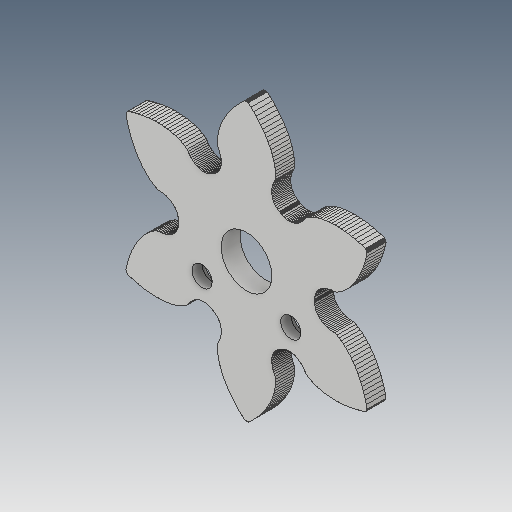
# Autodesk Inventor part: m5-6(dis0.4)
Saved by Autodesk Inventor 2019.4 (Build 234330000, 330)
## iProperties
Created: 2019-06-11
Part Number: m5-6(dis0.4)
Material: Generic
Document SubType Name: Modeling
Designer: AzLIer
Density: 1 g/cm^3
Appearance: Default
Mass: 2.28533 g
Surface Area: 21.9725 cm^2
Volume: 2.28533 cm^3
Autodesk Inventor part; units mm, degrees
ref_plane "YZ Plane" through (0, 0, 0) normal (1, 0, 0) x (0, 1, 0)
ref_plane "XZ Plane" through (0, 0, 0) normal (0, 1, 0) x (-1, 0, 0)
ref_plane "XY Plane" through (0, 0, 0) normal (0, 0, 1) x (1, 0, 0)
sketch "スケッチ1" plane through (0, 0, 0) normal (0, 0, 1) x (1, 0, 0)
  circle A0 centre (0, 0) radius 15 construction
  line L0 (-18, 0) -> (18, 0) construction
  line L1 (0, -18) -> (0, 18) construction
  line L2 (10.75, 0) -> (10.7499, 0.0461)
  line L3 (10.7499, 0.0461) -> (10.7496, 0.0922)
  line L4 (10.7496, 0.0922) -> (10.7491, 0.1384)
  line L5 (10.7491, 0.1384) -> (10.7484, 0.1845)
  line L6 (10.7484, 0.1845) -> (10.7475, 0.2306)
  line L7 (10.7475, 0.2306) -> (10.7652, 0.5329)
  line L8 (10.7652, 0.5329) -> (10.8097, 0.7549)
  line L9 (10.8097, 0.7549) -> (10.869, 0.9963)
  line L10 (10.869, 0.9963) -> (10.9454, 1.1976)
  line L11 (10.9454, 1.1976) -> (11.037, 1.3769)
  line L12 (11.037, 1.3769) -> (11.1429, 1.5397)
  line L13 (11.1429, 1.5397) -> (11.2607, 1.6996)
  line L14 (11.2607, 1.6996) -> (11.39, 1.856)
  line L15 (11.39, 1.856) -> (11.5328, 1.9955)
  line L16 (11.5328, 1.9955) -> (11.6888, 2.1189)
  line L17 (11.6888, 2.1189) -> (11.8558, 2.239)
  line L18 (11.8558, 2.239) -> (12.034, 2.3529)
  line L19 (12.034, 2.3529) -> (12.2259, 2.4472)
  line L20 (12.2259, 2.4472) -> (12.4297, 2.5309)
  line L21 (12.4297, 2.5309) -> (12.6434, 2.613)
  line L22 (12.6434, 2.613) -> (12.8716, 2.6699)
  line L23 (12.8716, 2.6699) -> (13.1096, 2.7237)
  line L24 (13.1096, 2.7237) -> (13.3595, 2.7636)
  line L25 (13.3595, 2.7636) -> (13.6235, 2.7775)
  line L26 (13.6235, 2.7775) -> (13.8941, 2.7998)
  line L27 (13.8941, 2.7998) -> (14.254, 2.9465)
  line L28 (14.254, 2.9465) -> (14.6036, 3.1397)
  line L29 (14.6036, 3.1397) -> (14.9447, 3.367)
  line L30 (14.9447, 3.367) -> (15.2773, 3.6237)
  line L31 (15.2773, 3.6237) -> (15.6013, 3.9073)
  line L32 (15.6013, 3.9073) -> (15.9161, 4.216)
  line L33 (15.9161, 4.216) -> (16.2214, 4.5483)
  line L34 (16.2214, 4.5483) -> (16.5165, 4.9034)
  line L35 (16.5165, 4.9034) -> (16.8007, 5.2802)
  line L36 (16.8007, 5.2802) -> (17.0734, 5.678)
  line L37 (17.0734, 5.678) -> (17.334, 6.0961)
  line L38 (17.334, 6.0961) -> (17.5819, 6.5338)
  line L39 (17.5819, 6.5338) -> (17.8162, 6.9906)
  line L40 (17.8162, 6.9906) -> (18.0365, 7.4658)
  line L41 (18.0365, 7.4658) -> (18.2419, 7.9587)
  line L42 (18.2419, 7.9587) -> (18.4319, 8.469)
  line L43 (18.4319, 8.469) -> (18.6058, 8.9958)
  line L44 (18.6058, 8.9958) -> (18.7629, 9.5386)
  line L45 (18.7629, 9.5386) -> (18.9026, 10.0969)
  line L46 (18.9026, 10.0969) -> (19.0243, 10.6699)
  line L47 (19.0243, 10.6699) -> (18.9976, 10.7173)
  line L48 (18.9976, 10.7173) -> (18.9709, 10.7646)
  line L49 (18.9709, 10.7646) -> (18.944, 10.8118)
  line L50 (18.944, 10.8118) -> (18.917, 10.859)
  line L51 (18.917, 10.859) -> (18.8899, 10.9061)
  line L52 (10.75, 0) -> (10.7499, -0.0461)
  line L53 (10.7499, -0.0461) -> (10.7496, -0.0922)
  line L54 (10.7496, -0.0922) -> (10.7491, -0.1384)
  line L55 (10.7491, -0.1384) -> (10.7484, -0.1845)
  line L56 (10.7484, -0.1845) -> (10.7475, -0.2306)
  line L57 (10.7475, -0.2306) -> (10.7652, -0.5329)
  line L58 (10.7652, -0.5329) -> (10.8097, -0.7549)
  line L59 (10.8097, -0.7549) -> (10.869, -0.9963)
  line L60 (10.869, -0.9963) -> (10.9454, -1.1976)
  line L61 (10.9454, -1.1976) -> (11.037, -1.3769)
  line L62 (11.037, -1.3769) -> (11.1429, -1.5397)
  line L63 (11.1429, -1.5397) -> (11.2607, -1.6996)
  line L64 (11.2607, -1.6996) -> (11.39, -1.856)
  line L65 (11.39, -1.856) -> (11.5328, -1.9955)
  line L66 (11.5328, -1.9955) -> (11.6888, -2.1189)
  line L67 (11.6888, -2.1189) -> (11.8558, -2.239)
  line L68 (11.8558, -2.239) -> (12.034, -2.3529)
  line L69 (12.034, -2.3529) -> (12.2259, -2.4472)
  line L70 (12.2259, -2.4472) -> (12.4297, -2.5309)
  line L71 (12.4297, -2.5309) -> (12.6434, -2.613)
  line L72 (12.6434, -2.613) -> (12.8716, -2.6699)
  line L73 (12.8716, -2.6699) -> (13.1096, -2.7237)
  line L74 (13.1096, -2.7237) -> (13.3595, -2.7636)
  line L75 (13.3595, -2.7636) -> (13.6235, -2.7775)
  line L76 (13.6235, -2.7775) -> (13.8941, -2.7998)
  line L77 (13.8941, -2.7998) -> (14.254, -2.9465)
  line L78 (14.254, -2.9465) -> (14.6036, -3.1397)
  line L79 (14.6036, -3.1397) -> (14.9447, -3.367)
  line L80 (14.9447, -3.367) -> (15.2773, -3.6237)
  line L81 (15.2773, -3.6237) -> (15.6013, -3.9073)
  line L82 (15.6013, -3.9073) -> (15.9161, -4.216)
  line L83 (15.9161, -4.216) -> (16.2214, -4.5483)
  line L84 (16.2214, -4.5483) -> (16.5165, -4.9034)
  line L85 (16.5165, -4.9034) -> (16.8007, -5.2802)
  line L86 (16.8007, -5.2802) -> (17.0734, -5.678)
  line L87 (17.0734, -5.678) -> (17.334, -6.0961)
  line L88 (17.334, -6.0961) -> (17.5819, -6.5338)
  line L89 (17.5819, -6.5338) -> (17.8162, -6.9906)
  line L90 (17.8162, -6.9906) -> (18.0365, -7.4658)
  line L91 (18.0365, -7.4658) -> (18.2419, -7.9587)
  line L92 (18.2419, -7.9587) -> (18.4319, -8.469)
  line L93 (18.4319, -8.469) -> (18.6058, -8.9958)
  line L94 (18.6058, -8.9958) -> (18.7629, -9.5386)
  line L95 (18.7629, -9.5386) -> (18.9026, -10.0969)
  line L96 (18.9026, -10.0969) -> (19.0243, -10.6699)
  line L97 (19.0243, -10.6699) -> (18.9976, -10.7173)
  line L98 (18.9976, -10.7173) -> (18.9709, -10.7646)
  line L99 (18.9709, -10.7646) -> (18.944, -10.8118)
  line L100 (18.944, -10.8118) -> (18.917, -10.859)
  line L101 (18.917, -10.859) -> (18.8899, -10.9061)
  line L102 (5.335, 9.3327) -> (5.2949, 9.3556)
  line L103 (5.2949, 9.3556) -> (5.2547, 9.3782)
  line L104 (4.238, 10.4198) -> (4.1585, 10.6018)
  line L105 (4.3261, 10.2467) -> (4.238, 10.4198)
  line L106 (4.4355, 10.0778) -> (4.3261, 10.2467)
  line L107 (4.5717, 9.9109) -> (4.4355, 10.0778)
  line L108 (4.751, 9.7389) -> (4.5717, 9.9109)
  line L109 (4.9211, 9.5894) -> (4.751, 9.7389)
  line L110 (5.1741, 9.4229) -> (4.9211, 9.5894)
  line L111 (5.2144, 9.4006) -> (5.1741, 9.4229)
  line L112 (5.2547, 9.3782) -> (5.2144, 9.4006)
  line L113 (4.1585, 10.6018) -> (4.0877, 10.792)
  line L114 (4.0877, 10.792) -> (4.0382, 10.9854)
  line L115 (4.0382, 10.9854) -> (4.0094, 11.1823)
  line L116 (4.0094, 11.1823) -> (3.9889, 11.3869)
  line L117 (3.9889, 11.3869) -> (3.9793, 11.5982)
  line L118 (3.9793, 11.5982) -> (3.9936, 11.8115)
  line L119 (3.9936, 11.8115) -> (4.023, 12.0299)
  line L120 (4.023, 12.0299) -> (4.0588, 12.2559)
  line L121 (4.1236, 12.4821) -> (4.196, 12.7151)
  line L122 (4.196, 12.7151) -> (4.2864, 12.9515)
  line L123 (4.2864, 12.9515) -> (4.4064, 13.187)
  line L124 (4.4064, 13.187) -> (4.5223, 13.4326)
  line L125 (4.5223, 13.4326) -> (4.5752, 13.8176)
  line L126 (4.5752, 13.8176) -> (4.5827, 14.217)
  line L127 (4.0588, 12.2559) -> (4.1236, 12.4821)
  line L128 (4.5827, 14.217) -> (4.5564, 14.626)
  line L129 (4.5564, 14.626) -> (4.5004, 15.0424)
  line L130 (4.5004, 15.0424) -> (4.4168, 15.4648)
  line L131 (4.4168, 15.4648) -> (4.3069, 15.8918)
  line L132 (4.3069, 15.8918) -> (4.1717, 16.3223)
  line L133 (4.1717, 16.3223) -> (4.0118, 16.7553)
  line L134 (4.0118, 16.7553) -> (3.8276, 17.1899)
  line L135 (3.8276, 17.1899) -> (3.6194, 17.625)
  line L136 (3.6194, 17.625) -> (3.3877, 18.0598)
  line L137 (3.3877, 18.0598) -> (3.1325, 18.4933)
  line L138 (3.1325, 18.4933) -> (2.8541, 18.9246)
  line L139 (2.8541, 18.9246) -> (2.5527, 19.3529)
  line L140 (2.5527, 19.3529) -> (2.2285, 19.7773)
  line L141 (2.2285, 19.7773) -> (1.8816, 20.197)
  line L142 (1.8816, 20.197) -> (1.5123, 20.611)
  line L143 (1.5123, 20.611) -> (1.1207, 21.0184)
  line L144 (1.1207, 21.0184) -> (0.7071, 21.4186)
  line L145 (0.2717, 21.8105) -> (0.2174, 21.8111)
  line L146 (0.2174, 21.8111) -> (0.163, 21.8116)
  line L147 (0.163, 21.8116) -> (0.1087, 21.8119)
  line L148 (0.1087, 21.8119) -> (0.0543, 21.8121)
  line L149 (0.0543, 21.8121) -> (0, 21.8122)
  line L150 (0.7071, 21.4186) -> (0.2717, 21.8105)
  line L151 (5.375, 9.3098) -> (5.335, 9.3327)
  line L152 (5.375, 9.3098) -> (5.4149, 9.2866)
  line L153 (5.4149, 9.2866) -> (5.4547, 9.2633)
  line L154 (5.4547, 9.2633) -> (5.4944, 9.2398)
  line L155 (5.4944, 9.2398) -> (5.534, 9.2162)
  line L156 (5.534, 9.2162) -> (5.5735, 9.1923)
  line L157 (5.5735, 9.1923) -> (5.8441, 9.0565)
  line L158 (5.8441, 9.0565) -> (6.0586, 8.984)
  line L159 (6.2973, 8.9146) -> (6.5098, 8.8802)
  line L160 (6.5098, 8.8802) -> (6.7109, 8.8699)
  line L161 (6.7109, 8.8699) -> (6.9048, 8.8802)
  line L162 (6.0586, 8.984) -> (6.2973, 8.9146)
  line L163 (6.9048, 8.8802) -> (7.1022, 8.9022)
  line L164 (7.1022, 8.9022) -> (7.3024, 8.936)
  line L165 (7.3024, 8.936) -> (7.4945, 8.9899)
  line L166 (7.4945, 8.9899) -> (7.6794, 9.0634)
  line L167 (7.6794, 9.0634) -> (7.8669, 9.1479)
  line L168 (7.8669, 9.1479) -> (8.0546, 9.2453)
  line L169 (8.0546, 9.2453) -> (8.2323, 9.3643)
  line L170 (8.2323, 9.3643) -> (8.4067, 9.499)
  line L171 (8.4067, 9.499) -> (8.5846, 9.643)
  line L172 (8.5846, 9.643) -> (8.748, 9.8122)
  line L173 (8.748, 9.8122) -> (8.9136, 9.9914)
  line L174 (8.9136, 9.9914) -> (9.0731, 10.1878)
  line L175 (9.2171, 10.4095) -> (9.3718, 10.6328)
  line L176 (9.3718, 10.6328) -> (9.6788, 10.8711)
  line L177 (9.0731, 10.1878) -> (9.2171, 10.4095)
  line L178 (9.6788, 10.8711) -> (10.0209, 11.0772)
  line L179 (10.0209, 11.0772) -> (10.3882, 11.259)
  line L180 (10.3882, 11.259) -> (10.7769, 11.4187)
  line L181 (10.7769, 11.4187) -> (11.1845, 11.5574)
  line L182 (11.1845, 11.5574) -> (11.6092, 11.6758)
  line L183 (11.6092, 11.6758) -> (12.0497, 11.774)
  line L184 (12.0497, 11.774) -> (12.5047, 11.852)
  line L185 (17.0935, 11.6152) -> (17.6421, 11.4798)
  line L186 (17.6421, 11.4798) -> (18.1955, 11.3217)
  line L187 (18.1955, 11.3217) -> (18.7526, 11.1405)
  line L188 (18.7526, 11.1405) -> (18.7803, 11.0938)
  line L189 (18.7803, 11.0938) -> (18.8079, 11.047)
  line L190 (18.8079, 11.047) -> (18.8353, 11.0001)
  line L191 (18.8353, 11.0001) -> (18.8627, 10.9531)
  line L192 (18.8627, 10.9531) -> (18.8899, 10.9061)
  line L193 (12.9731, 11.9097) -> (13.454, 11.947)
  line L194 (13.454, 11.947) -> (13.9464, 11.9637)
  line L195 (13.9464, 11.9637) -> (14.4494, 11.9594)
  line L196 (14.4494, 11.9594) -> (14.9621, 11.934)
  line L197 (14.9621, 11.934) -> (15.4838, 11.8872)
  line L198 (15.4838, 11.8872) -> (16.0134, 11.8186)
  line L199 (16.0134, 11.8186) -> (16.5503, 11.728)
  line L200 (16.5503, 11.728) -> (17.0935, 11.6152)
  line L201 (12.5047, 11.852) -> (12.9731, 11.9097)
  line L202 (-5.4149, 9.2866) -> (-5.4547, 9.2633)
  line L203 (-5.4547, 9.2633) -> (-5.4944, 9.2398)
  line L204 (-6.9048, 8.8802) -> (-7.1022, 8.9022)
  line L205 (-6.7109, 8.8699) -> (-6.9048, 8.8802)
  line L206 (-6.5098, 8.8802) -> (-6.7109, 8.8699)
  line L207 (-6.2973, 8.9146) -> (-6.5098, 8.8802)
  line L208 (-6.0586, 8.984) -> (-6.2973, 8.9146)
  line L209 (-5.8441, 9.0565) -> (-6.0586, 8.984)
  line L210 (-5.5735, 9.1923) -> (-5.8441, 9.0565)
  line L211 (-5.534, 9.2162) -> (-5.5735, 9.1923)
  line L212 (-5.4944, 9.2398) -> (-5.534, 9.2162)
  line L213 (-7.1022, 8.9022) -> (-7.3024, 8.936)
  line L214 (-7.3024, 8.936) -> (-7.4945, 8.9899)
  line L215 (-7.4945, 8.9899) -> (-7.6794, 9.0634)
  line L216 (-7.6794, 9.0634) -> (-7.8669, 9.1479)
  line L217 (-7.8669, 9.1479) -> (-8.0546, 9.2453)
  line L218 (-8.0546, 9.2453) -> (-8.2323, 9.3643)
  line L219 (-8.2323, 9.3643) -> (-8.4067, 9.499)
  line L220 (-8.4067, 9.499) -> (-8.5846, 9.643)
  line L221 (-8.748, 9.8122) -> (-8.9136, 9.9914)
  line L222 (-8.9136, 9.9914) -> (-9.0731, 10.1878)
  line L223 (-9.0731, 10.1878) -> (-9.2171, 10.4095)
  line L224 (-9.2171, 10.4095) -> (-9.3718, 10.6328)
  line L225 (-9.3718, 10.6328) -> (-9.6788, 10.8711)
  line L226 (-9.6788, 10.8711) -> (-10.0209, 11.0772)
  line L227 (-8.5846, 9.643) -> (-8.748, 9.8122)
  line L228 (-10.0209, 11.0772) -> (-10.3882, 11.259)
  line L229 (-10.3882, 11.259) -> (-10.7769, 11.4187)
  line L230 (-10.7769, 11.4187) -> (-11.1845, 11.5574)
  line L231 (-11.1845, 11.5574) -> (-11.6092, 11.6758)
  line L232 (-11.6092, 11.6758) -> (-12.0497, 11.774)
  line L233 (-12.0497, 11.774) -> (-12.5047, 11.852)
  line L234 (-12.5047, 11.852) -> (-12.9731, 11.9097)
  line L235 (-12.9731, 11.9097) -> (-13.454, 11.947)
  line L236 (-13.454, 11.947) -> (-13.9464, 11.9637)
  line L237 (-13.9464, 11.9637) -> (-14.4494, 11.9594)
  line L238 (-14.4494, 11.9594) -> (-14.9621, 11.934)
  line L239 (-14.9621, 11.934) -> (-15.4838, 11.8872)
  line L240 (-15.4838, 11.8872) -> (-16.0134, 11.8186)
  line L241 (-16.0134, 11.8186) -> (-16.5503, 11.728)
  line L242 (-16.5503, 11.728) -> (-17.0935, 11.6152)
  line L243 (-17.0935, 11.6152) -> (-17.6421, 11.4798)
  line L244 (-17.6421, 11.4798) -> (-18.1955, 11.3217)
  line L245 (-18.7526, 11.1405) -> (-18.7803, 11.0938)
  line L246 (-18.7803, 11.0938) -> (-18.8079, 11.047)
  line L247 (-18.8079, 11.047) -> (-18.8353, 11.0001)
  line L248 (-18.8353, 11.0001) -> (-18.8627, 10.9531)
  line L249 (-18.8627, 10.9531) -> (-18.8899, 10.9061)
  line L250 (-18.1955, 11.3217) -> (-18.7526, 11.1405)
  line L251 (-5.375, 9.3098) -> (-5.4149, 9.2866)
  line L252 (-5.375, 9.3098) -> (-5.335, 9.3327)
  line L253 (-5.335, 9.3327) -> (-5.2949, 9.3556)
  line L254 (-5.2949, 9.3556) -> (-5.2547, 9.3782)
  line L255 (-5.2547, 9.3782) -> (-5.2144, 9.4006)
  line L256 (-5.2144, 9.4006) -> (-5.1741, 9.4229)
  line L257 (-5.1741, 9.4229) -> (-4.9211, 9.5894)
  line L258 (-4.9211, 9.5894) -> (-4.751, 9.7389)
  line L259 (-4.5717, 9.9109) -> (-4.4355, 10.0778)
  line L260 (-4.4355, 10.0778) -> (-4.3261, 10.2467)
  line L261 (-4.3261, 10.2467) -> (-4.238, 10.4198)
  line L262 (-4.751, 9.7389) -> (-4.5717, 9.9109)
  line L263 (-4.238, 10.4198) -> (-4.1585, 10.6018)
  line L264 (-4.1585, 10.6018) -> (-4.0877, 10.792)
  line L265 (-4.0877, 10.792) -> (-4.0382, 10.9854)
  line L266 (-4.0382, 10.9854) -> (-4.0094, 11.1823)
  line L267 (-4.0094, 11.1823) -> (-3.9889, 11.3869)
  line L268 (-3.9889, 11.3869) -> (-3.9793, 11.5982)
  line L269 (-3.9793, 11.5982) -> (-3.9936, 11.8115)
  line L270 (-3.9936, 11.8115) -> (-4.023, 12.0299)
  line L271 (-4.023, 12.0299) -> (-4.0588, 12.2559)
  line L272 (-4.0588, 12.2559) -> (-4.1236, 12.4821)
  line L273 (-4.1236, 12.4821) -> (-4.196, 12.7151)
  line L274 (-4.196, 12.7151) -> (-4.2864, 12.9515)
  line L275 (-4.4064, 13.187) -> (-4.5223, 13.4326)
  line L276 (-4.5223, 13.4326) -> (-4.5752, 13.8176)
  line L277 (-4.2864, 12.9515) -> (-4.4064, 13.187)
  line L278 (-4.5752, 13.8176) -> (-4.5827, 14.217)
  line L279 (-4.5827, 14.217) -> (-4.5564, 14.626)
  line L280 (-4.5564, 14.626) -> (-4.5004, 15.0424)
  line L281 (-4.5004, 15.0424) -> (-4.4168, 15.4648)
  line L282 (-4.4168, 15.4648) -> (-4.3069, 15.8918)
  line L283 (-4.3069, 15.8918) -> (-4.1717, 16.3223)
  line L284 (-4.1717, 16.3223) -> (-4.0118, 16.7553)
  line L285 (-1.5123, 20.611) -> (-1.1207, 21.0184)
  line L286 (-1.1207, 21.0184) -> (-0.7071, 21.4186)
  line L287 (-0.7071, 21.4186) -> (-0.2717, 21.8105)
  line L288 (-0.2717, 21.8105) -> (-0.2174, 21.8111)
  line L289 (-0.2174, 21.8111) -> (-0.163, 21.8116)
  line L290 (-0.163, 21.8116) -> (-0.1087, 21.8119)
  line L291 (-0.1087, 21.8119) -> (-0.0543, 21.8121)
  line L292 (-0.0543, 21.8121) -> (0, 21.8122)
  line L293 (-3.8276, 17.1899) -> (-3.6194, 17.625)
  line L294 (-3.6194, 17.625) -> (-3.3877, 18.0598)
  line L295 (-3.3877, 18.0598) -> (-3.1325, 18.4933)
  line L296 (-3.1325, 18.4933) -> (-2.8541, 18.9246)
  line L297 (-2.8541, 18.9246) -> (-2.5527, 19.3529)
  line L298 (-2.5527, 19.3529) -> (-2.2285, 19.7773)
  line L299 (-2.2285, 19.7773) -> (-1.8816, 20.197)
  line L300 (-1.8816, 20.197) -> (-1.5123, 20.611)
  line L301 (-4.0118, 16.7553) -> (-3.8276, 17.1899)
  line L302 (-10.7499, -0.0461) -> (-10.7496, -0.0922)
  line L303 (-10.7496, -0.0922) -> (-10.7491, -0.1384)
  line L304 (-11.1429, -1.5397) -> (-11.2607, -1.6996)
  line L305 (-11.037, -1.3769) -> (-11.1429, -1.5397)
  line L306 (-10.9454, -1.1976) -> (-11.037, -1.3769)
  line L307 (-10.869, -0.9963) -> (-10.9454, -1.1976)
  line L308 (-10.8097, -0.7549) -> (-10.869, -0.9963)
  line L309 (-10.7652, -0.5329) -> (-10.8097, -0.7549)
  line L310 (-10.7475, -0.2306) -> (-10.7652, -0.5329)
  line L311 (-10.7484, -0.1845) -> (-10.7475, -0.2306)
  line L312 (-10.7491, -0.1384) -> (-10.7484, -0.1845)
  line L313 (-11.2607, -1.6996) -> (-11.39, -1.856)
  line L314 (-11.39, -1.856) -> (-11.5328, -1.9955)
  line L315 (-11.5328, -1.9955) -> (-11.6888, -2.1189)
  line L316 (-11.6888, -2.1189) -> (-11.8558, -2.239)
  line L317 (-11.8558, -2.239) -> (-12.034, -2.3529)
  line L318 (-12.034, -2.3529) -> (-12.2259, -2.4472)
  line L319 (-12.2259, -2.4472) -> (-12.4297, -2.5309)
  line L320 (-12.4297, -2.5309) -> (-12.6434, -2.613)
  line L321 (-12.8716, -2.6699) -> (-13.1096, -2.7237)
  line L322 (-13.1096, -2.7237) -> (-13.3595, -2.7636)
  line L323 (-13.3595, -2.7636) -> (-13.6235, -2.7775)
  line L324 (-13.6235, -2.7775) -> (-13.8941, -2.7998)
  line L325 (-13.8941, -2.7998) -> (-14.254, -2.9465)
  line L326 (-14.254, -2.9465) -> (-14.6036, -3.1397)
  line L327 (-12.6434, -2.613) -> (-12.8716, -2.6699)
  line L328 (-14.6036, -3.1397) -> (-14.9447, -3.367)
  line L329 (-14.9447, -3.367) -> (-15.2773, -3.6237)
  line L330 (-15.2773, -3.6237) -> (-15.6013, -3.9073)
  line L331 (-15.6013, -3.9073) -> (-15.9161, -4.216)
  line L332 (-15.9161, -4.216) -> (-16.2214, -4.5483)
  line L333 (-16.2214, -4.5483) -> (-16.5165, -4.9034)
  line L334 (-16.5165, -4.9034) -> (-16.8007, -5.2802)
  line L335 (-16.8007, -5.2802) -> (-17.0734, -5.678)
  line L336 (-17.0734, -5.678) -> (-17.334, -6.0961)
  line L337 (-17.334, -6.0961) -> (-17.5819, -6.5338)
  line L338 (-17.5819, -6.5338) -> (-17.8162, -6.9906)
  line L339 (-17.8162, -6.9906) -> (-18.0365, -7.4658)
  line L340 (-18.0365, -7.4658) -> (-18.2419, -7.9587)
  line L341 (-18.2419, -7.9587) -> (-18.4319, -8.469)
  line L342 (-18.4319, -8.469) -> (-18.6058, -8.9958)
  line L343 (-18.6058, -8.9958) -> (-18.7629, -9.5386)
  line L344 (-18.7629, -9.5386) -> (-18.9026, -10.0969)
  line L345 (-19.0243, -10.6699) -> (-18.9976, -10.7173)
  line L346 (-18.9976, -10.7173) -> (-18.9709, -10.7646)
  line L347 (-18.9709, -10.7646) -> (-18.944, -10.8118)
  line L348 (-18.944, -10.8118) -> (-18.917, -10.859)
  line L349 (-18.917, -10.859) -> (-18.8899, -10.9061)
  line L350 (-18.9026, -10.0969) -> (-19.0243, -10.6699)
  line L351 (-10.75, 0) -> (-10.7499, -0.0461)
  line L352 (-10.75, 0) -> (-10.7499, 0.0461)
  line L353 (-10.7499, 0.0461) -> (-10.7496, 0.0922)
  line L354 (-10.7496, 0.0922) -> (-10.7491, 0.1384)
  line L355 (-10.7491, 0.1384) -> (-10.7484, 0.1845)
  line L356 (-10.7484, 0.1845) -> (-10.7475, 0.2306)
  line L357 (-10.7475, 0.2306) -> (-10.7652, 0.5329)
  line L358 (-10.7652, 0.5329) -> (-10.8097, 0.7549)
  line L359 (-10.869, 0.9963) -> (-10.9454, 1.1976)
  line L360 (-10.9454, 1.1976) -> (-11.037, 1.3769)
  line L361 (-11.037, 1.3769) -> (-11.1429, 1.5397)
  line L362 (-10.8097, 0.7549) -> (-10.869, 0.9963)
  line L363 (-11.1429, 1.5397) -> (-11.2607, 1.6996)
  line L364 (-11.2607, 1.6996) -> (-11.39, 1.856)
  line L365 (-11.39, 1.856) -> (-11.5328, 1.9955)
  line L366 (-11.5328, 1.9955) -> (-11.6888, 2.1189)
  line L367 (-11.6888, 2.1189) -> (-11.8558, 2.239)
  line L368 (-11.8558, 2.239) -> (-12.034, 2.3529)
  line L369 (-12.034, 2.3529) -> (-12.2259, 2.4472)
  line L370 (-12.2259, 2.4472) -> (-12.4297, 2.5309)
  line L371 (-12.4297, 2.5309) -> (-12.6434, 2.613)
  line L372 (-12.6434, 2.613) -> (-12.8716, 2.6699)
  line L373 (-12.8716, 2.6699) -> (-13.1096, 2.7237)
  line L374 (-13.1096, 2.7237) -> (-13.3595, 2.7636)
  line L375 (-13.6235, 2.7775) -> (-13.8941, 2.7998)
  line L376 (-13.8941, 2.7998) -> (-14.254, 2.9465)
  line L377 (-13.3595, 2.7636) -> (-13.6235, 2.7775)
  line L378 (-14.254, 2.9465) -> (-14.6036, 3.1397)
  line L379 (-14.6036, 3.1397) -> (-14.9447, 3.367)
  line L380 (-14.9447, 3.367) -> (-15.2773, 3.6237)
  line L381 (-15.2773, 3.6237) -> (-15.6013, 3.9073)
  line L382 (-15.6013, 3.9073) -> (-15.9161, 4.216)
  line L383 (-15.9161, 4.216) -> (-16.2214, 4.5483)
  line L384 (-16.2214, 4.5483) -> (-16.5165, 4.9034)
  line L385 (-18.6058, 8.9958) -> (-18.7629, 9.5386)
  line L386 (-18.7629, 9.5386) -> (-18.9026, 10.0969)
  line L387 (-18.9026, 10.0969) -> (-19.0243, 10.6699)
  line L388 (-19.0243, 10.6699) -> (-18.9976, 10.7173)
  line L389 (-18.9976, 10.7173) -> (-18.9709, 10.7646)
  line L390 (-18.9709, 10.7646) -> (-18.944, 10.8118)
  line L391 (-18.944, 10.8118) -> (-18.917, 10.859)
  line L392 (-18.917, 10.859) -> (-18.8899, 10.9061)
  line L393 (-16.8007, 5.2802) -> (-17.0734, 5.678)
  line L394 (-17.0734, 5.678) -> (-17.334, 6.0961)
  line L395 (-17.334, 6.0961) -> (-17.5819, 6.5338)
  line L396 (-17.5819, 6.5338) -> (-17.8162, 6.9906)
  line L397 (-17.8162, 6.9906) -> (-18.0365, 7.4658)
  line L398 (-18.0365, 7.4658) -> (-18.2419, 7.9587)
  line L399 (-18.2419, 7.9587) -> (-18.4319, 8.469)
  line L400 (-18.4319, 8.469) -> (-18.6058, 8.9958)
  line L401 (-16.5165, 4.9034) -> (-16.8007, 5.2802)
  line L402 (-5.335, -9.3327) -> (-5.2949, -9.3556)
  line L403 (-5.2949, -9.3556) -> (-5.2547, -9.3782)
  line L404 (-4.238, -10.4198) -> (-4.1585, -10.6018)
  line L405 (-4.3261, -10.2467) -> (-4.238, -10.4198)
  line L406 (-4.4355, -10.0778) -> (-4.3261, -10.2467)
  line L407 (-4.5717, -9.9109) -> (-4.4355, -10.0778)
  line L408 (-4.751, -9.7389) -> (-4.5717, -9.9109)
  line L409 (-4.9211, -9.5894) -> (-4.751, -9.7389)
  line L410 (-5.1741, -9.4229) -> (-4.9211, -9.5894)
  line L411 (-5.2144, -9.4006) -> (-5.1741, -9.4229)
  line L412 (-5.2547, -9.3782) -> (-5.2144, -9.4006)
  line L413 (-4.1585, -10.6018) -> (-4.0877, -10.792)
  line L414 (-4.0877, -10.792) -> (-4.0382, -10.9854)
  line L415 (-4.0382, -10.9854) -> (-4.0094, -11.1823)
  line L416 (-4.0094, -11.1823) -> (-3.9889, -11.3869)
  line L417 (-3.9889, -11.3869) -> (-3.9793, -11.5982)
  line L418 (-3.9793, -11.5982) -> (-3.9936, -11.8115)
  line L419 (-3.9936, -11.8115) -> (-4.023, -12.0299)
  line L420 (-4.023, -12.0299) -> (-4.0588, -12.2559)
  line L421 (-4.1236, -12.4821) -> (-4.196, -12.7151)
  line L422 (-4.196, -12.7151) -> (-4.2864, -12.9515)
  line L423 (-4.2864, -12.9515) -> (-4.4064, -13.187)
  line L424 (-4.4064, -13.187) -> (-4.5223, -13.4326)
  line L425 (-4.5223, -13.4326) -> (-4.5752, -13.8176)
  line L426 (-4.5752, -13.8176) -> (-4.5827, -14.217)
  line L427 (-4.0588, -12.2559) -> (-4.1236, -12.4821)
  line L428 (-4.5827, -14.217) -> (-4.5564, -14.626)
  line L429 (-4.5564, -14.626) -> (-4.5004, -15.0424)
  line L430 (-4.5004, -15.0424) -> (-4.4168, -15.4648)
  line L431 (-4.4168, -15.4648) -> (-4.3069, -15.8918)
  line L432 (-4.3069, -15.8918) -> (-4.1717, -16.3223)
  line L433 (-4.1717, -16.3223) -> (-4.0118, -16.7553)
  line L434 (-4.0118, -16.7553) -> (-3.8276, -17.1899)
  line L435 (-3.8276, -17.1899) -> (-3.6194, -17.625)
  line L436 (-3.6194, -17.625) -> (-3.3877, -18.0598)
  line L437 (-3.3877, -18.0598) -> (-3.1325, -18.4933)
  line L438 (-3.1325, -18.4933) -> (-2.8541, -18.9246)
  line L439 (-2.8541, -18.9246) -> (-2.5527, -19.3529)
  line L440 (-2.5527, -19.3529) -> (-2.2285, -19.7773)
  line L441 (-2.2285, -19.7773) -> (-1.8816, -20.197)
  line L442 (-1.8816, -20.197) -> (-1.5123, -20.611)
  line L443 (-1.5123, -20.611) -> (-1.1207, -21.0184)
  line L444 (-1.1207, -21.0184) -> (-0.7071, -21.4186)
  line L445 (-0.2717, -21.8105) -> (-0.2174, -21.8111)
  line L446 (-0.2174, -21.8111) -> (-0.163, -21.8116)
  line L447 (-0.163, -21.8116) -> (-0.1087, -21.8119)
  line L448 (-0.1087, -21.8119) -> (-0.0543, -21.8121)
  line L449 (-0.0543, -21.8121) -> (0, -21.8122)
  line L450 (-0.7071, -21.4186) -> (-0.2717, -21.8105)
  line L451 (-5.375, -9.3098) -> (-5.335, -9.3327)
  line L452 (-5.375, -9.3098) -> (-5.4149, -9.2866)
  line L453 (-5.4149, -9.2866) -> (-5.4547, -9.2633)
  line L454 (-5.4547, -9.2633) -> (-5.4944, -9.2398)
  line L455 (-5.4944, -9.2398) -> (-5.534, -9.2162)
  line L456 (-5.534, -9.2162) -> (-5.5735, -9.1923)
  line L457 (-5.5735, -9.1923) -> (-5.8441, -9.0565)
  line L458 (-5.8441, -9.0565) -> (-6.0586, -8.984)
  line L459 (-6.2973, -8.9146) -> (-6.5098, -8.8802)
  line L460 (-6.5098, -8.8802) -> (-6.7109, -8.8699)
  line L461 (-6.7109, -8.8699) -> (-6.9048, -8.8802)
  line L462 (-6.0586, -8.984) -> (-6.2973, -8.9146)
  line L463 (-6.9048, -8.8802) -> (-7.1022, -8.9022)
  line L464 (-7.1022, -8.9022) -> (-7.3024, -8.936)
  line L465 (-7.3024, -8.936) -> (-7.4945, -8.9899)
  line L466 (-7.4945, -8.9899) -> (-7.6794, -9.0634)
  line L467 (-7.6794, -9.0634) -> (-7.8669, -9.1479)
  line L468 (-7.8669, -9.1479) -> (-8.0546, -9.2453)
  line L469 (-8.0546, -9.2453) -> (-8.2323, -9.3643)
  line L470 (-8.2323, -9.3643) -> (-8.4067, -9.499)
  line L471 (-8.4067, -9.499) -> (-8.5846, -9.643)
  line L472 (-8.5846, -9.643) -> (-8.748, -9.8122)
  line L473 (-8.748, -9.8122) -> (-8.9136, -9.9914)
  line L474 (-8.9136, -9.9914) -> (-9.0731, -10.1878)
  line L475 (-9.2171, -10.4095) -> (-9.3718, -10.6328)
  line L476 (-9.3718, -10.6328) -> (-9.6788, -10.8711)
  line L477 (-9.0731, -10.1878) -> (-9.2171, -10.4095)
  line L478 (-9.6788, -10.8711) -> (-10.0209, -11.0772)
  line L479 (-10.0209, -11.0772) -> (-10.3882, -11.259)
  line L480 (-10.3882, -11.259) -> (-10.7769, -11.4187)
  line L481 (-10.7769, -11.4187) -> (-11.1845, -11.5574)
  line L482 (-11.1845, -11.5574) -> (-11.6092, -11.6758)
  line L483 (-11.6092, -11.6758) -> (-12.0497, -11.774)
  line L484 (-12.0497, -11.774) -> (-12.5047, -11.852)
  line L485 (-17.0935, -11.6152) -> (-17.6421, -11.4798)
  line L486 (-17.6421, -11.4798) -> (-18.1955, -11.3217)
  line L487 (-18.1955, -11.3217) -> (-18.7526, -11.1405)
  line L488 (-18.7526, -11.1405) -> (-18.7803, -11.0938)
  line L489 (-18.7803, -11.0938) -> (-18.8079, -11.047)
  line L490 (-18.8079, -11.047) -> (-18.8353, -11.0001)
  line L491 (-18.8353, -11.0001) -> (-18.8627, -10.9531)
  line L492 (-18.8627, -10.9531) -> (-18.8899, -10.9061)
  line L493 (-12.9731, -11.9097) -> (-13.454, -11.947)
  line L494 (-13.454, -11.947) -> (-13.9464, -11.9637)
  line L495 (-13.9464, -11.9637) -> (-14.4494, -11.9594)
  line L496 (-14.4494, -11.9594) -> (-14.9621, -11.934)
  line L497 (-14.9621, -11.934) -> (-15.4838, -11.8872)
  line L498 (-15.4838, -11.8872) -> (-16.0134, -11.8186)
  line L499 (-16.0134, -11.8186) -> (-16.5503, -11.728)
  line L500 (-16.5503, -11.728) -> (-17.0935, -11.6152)
  line L501 (-12.5047, -11.852) -> (-12.9731, -11.9097)
  line L502 (5.4149, -9.2866) -> (5.4547, -9.2633)
  line L503 (5.4547, -9.2633) -> (5.4944, -9.2398)
  line L504 (6.9048, -8.8802) -> (7.1022, -8.9022)
  line L505 (6.7109, -8.8699) -> (6.9048, -8.8802)
  line L506 (6.5098, -8.8802) -> (6.7109, -8.8699)
  line L507 (6.2973, -8.9146) -> (6.5098, -8.8802)
  line L508 (6.0586, -8.984) -> (6.2973, -8.9146)
  line L509 (5.8441, -9.0565) -> (6.0586, -8.984)
  line L510 (5.5735, -9.1923) -> (5.8441, -9.0565)
  line L511 (5.534, -9.2162) -> (5.5735, -9.1923)
  line L512 (5.4944, -9.2398) -> (5.534, -9.2162)
  line L513 (7.1022, -8.9022) -> (7.3024, -8.936)
  line L514 (7.3024, -8.936) -> (7.4945, -8.9899)
  line L515 (7.4945, -8.9899) -> (7.6794, -9.0634)
  line L516 (7.6794, -9.0634) -> (7.8669, -9.1479)
  line L517 (7.8669, -9.1479) -> (8.0546, -9.2453)
  line L518 (8.0546, -9.2453) -> (8.2323, -9.3643)
  line L519 (8.2323, -9.3643) -> (8.4067, -9.499)
  line L520 (8.4067, -9.499) -> (8.5846, -9.643)
  line L521 (8.748, -9.8122) -> (8.9136, -9.9914)
  line L522 (8.9136, -9.9914) -> (9.0731, -10.1878)
  line L523 (9.0731, -10.1878) -> (9.2171, -10.4095)
  line L524 (9.2171, -10.4095) -> (9.3718, -10.6328)
  line L525 (9.3718, -10.6328) -> (9.6788, -10.8711)
  line L526 (9.6788, -10.8711) -> (10.0209, -11.0772)
  line L527 (8.5846, -9.643) -> (8.748, -9.8122)
  line L528 (10.0209, -11.0772) -> (10.3882, -11.259)
  line L529 (10.3882, -11.259) -> (10.7769, -11.4187)
  line L530 (10.7769, -11.4187) -> (11.1845, -11.5574)
  line L531 (11.1845, -11.5574) -> (11.6092, -11.6758)
  line L532 (11.6092, -11.6758) -> (12.0497, -11.774)
  line L533 (12.0497, -11.774) -> (12.5047, -11.852)
  line L534 (12.5047, -11.852) -> (12.9731, -11.9097)
  line L535 (12.9731, -11.9097) -> (13.454, -11.947)
  line L536 (13.454, -11.947) -> (13.9464, -11.9637)
  line L537 (13.9464, -11.9637) -> (14.4494, -11.9594)
  line L538 (14.4494, -11.9594) -> (14.9621, -11.934)
  line L539 (14.9621, -11.934) -> (15.4838, -11.8872)
  line L540 (15.4838, -11.8872) -> (16.0134, -11.8186)
  line L541 (16.0134, -11.8186) -> (16.5503, -11.728)
  line L542 (16.5503, -11.728) -> (17.0935, -11.6152)
  line L543 (17.0935, -11.6152) -> (17.6421, -11.4798)
  line L544 (17.6421, -11.4798) -> (18.1955, -11.3217)
  line L545 (18.7526, -11.1405) -> (18.7803, -11.0938)
  line L546 (18.7803, -11.0938) -> (18.8079, -11.047)
  line L547 (18.8079, -11.047) -> (18.8353, -11.0001)
  line L548 (18.8353, -11.0001) -> (18.8627, -10.9531)
  line L549 (18.8627, -10.9531) -> (18.8899, -10.9061)
  line L550 (18.1955, -11.3217) -> (18.7526, -11.1405)
  line L551 (5.375, -9.3098) -> (5.4149, -9.2866)
  line L552 (5.375, -9.3098) -> (5.335, -9.3327)
  line L553 (5.335, -9.3327) -> (5.2949, -9.3556)
  line L554 (5.2949, -9.3556) -> (5.2547, -9.3782)
  line L555 (5.2547, -9.3782) -> (5.2144, -9.4006)
  line L556 (5.2144, -9.4006) -> (5.1741, -9.4229)
  line L557 (5.1741, -9.4229) -> (4.9211, -9.5894)
  line L558 (4.9211, -9.5894) -> (4.751, -9.7389)
  line L559 (4.5717, -9.9109) -> (4.4355, -10.0778)
  line L560 (4.4355, -10.0778) -> (4.3261, -10.2467)
  line L561 (4.3261, -10.2467) -> (4.238, -10.4198)
  line L562 (4.751, -9.7389) -> (4.5717, -9.9109)
  line L563 (4.238, -10.4198) -> (4.1585, -10.6018)
  line L564 (4.1585, -10.6018) -> (4.0877, -10.792)
  line L565 (4.0877, -10.792) -> (4.0382, -10.9854)
  line L566 (4.0382, -10.9854) -> (4.0094, -11.1823)
  line L567 (4.0094, -11.1823) -> (3.9889, -11.3869)
  line L568 (3.9889, -11.3869) -> (3.9793, -11.5982)
  line L569 (3.9793, -11.5982) -> (3.9936, -11.8115)
  line L570 (3.9936, -11.8115) -> (4.023, -12.0299)
  line L571 (4.023, -12.0299) -> (4.0588, -12.2559)
  line L572 (4.0588, -12.2559) -> (4.1236, -12.4821)
  line L573 (4.1236, -12.4821) -> (4.196, -12.7151)
  line L574 (4.196, -12.7151) -> (4.2864, -12.9515)
  line L575 (4.4064, -13.187) -> (4.5223, -13.4326)
  line L576 (4.5223, -13.4326) -> (4.5752, -13.8176)
  line L577 (4.2864, -12.9515) -> (4.4064, -13.187)
  line L578 (4.5752, -13.8176) -> (4.5827, -14.217)
  line L579 (4.5827, -14.217) -> (4.5564, -14.626)
  line L580 (4.5564, -14.626) -> (4.5004, -15.0424)
  line L581 (4.5004, -15.0424) -> (4.4168, -15.4648)
  line L582 (4.4168, -15.4648) -> (4.3069, -15.8918)
  line L583 (4.3069, -15.8918) -> (4.1717, -16.3223)
  line L584 (4.1717, -16.3223) -> (4.0118, -16.7553)
  line L585 (1.5123, -20.611) -> (1.1207, -21.0184)
  line L586 (1.1207, -21.0184) -> (0.7071, -21.4186)
  line L587 (0.7071, -21.4186) -> (0.2717, -21.8105)
  line L588 (0.2717, -21.8105) -> (0.2174, -21.8111)
  line L589 (0.2174, -21.8111) -> (0.163, -21.8116)
  line L590 (0.163, -21.8116) -> (0.1087, -21.8119)
  line L591 (0.1087, -21.8119) -> (0.0543, -21.8121)
  line L592 (0.0543, -21.8121) -> (0, -21.8122)
  line L593 (3.8276, -17.1899) -> (3.6194, -17.625)
  line L594 (3.6194, -17.625) -> (3.3877, -18.0598)
  line L595 (3.3877, -18.0598) -> (3.1325, -18.4933)
  line L596 (3.1325, -18.4933) -> (2.8541, -18.9246)
  line L597 (2.8541, -18.9246) -> (2.5527, -19.3529)
  line L598 (2.5527, -19.3529) -> (2.2285, -19.7773)
  line L599 (2.2285, -19.7773) -> (1.8816, -20.197)
  line L600 (1.8816, -20.197) -> (1.5123, -20.611)
  line L601 (4.0118, -16.7553) -> (3.8276, -17.1899)
  circle A1 centre (0, 0) radius 4
  dimension "d6" = 8
  constraints: 1204 end point, 50 symmetric about line, 2 centre point, 1 coincident, 1 point on line
  measures "d6" diameter of A1
extrude "押し出し1" add sketch "スケッチ1" along normal blind 3
sketch "スケッチ2" plane through (0, 0, 0) normal (0, 0, -1) x (-1, 0, 0)
  line L0 (-10, -8) -> (10, -8)
  line L1 (10, -8) -> (10, -3)
  line L2 (10, -3) -> (-10, -3)
  line L3 (-10, -3) -> (-10, -8)
  line L4 (-10, -8) -> (10, -3) construction
  line L5 (10, -8) -> (-10, -3) construction
  line L6 (7, -5.5) -> (-7, -5.5)
  point P0 (0, 0)
  point P1 (0, -5.5)
  point P2 (0, -5.5)
  dimension "d8" = 3
  dimension "d9" = 5
  dimension "d10" = 20
  dimension "d11" = 14
  constraints: 14 end point, 4 midpoint, 2 horizontal, 2 parallel, 1 perpendicular, 1 vertical alignment
  measures "d8" distance from line of point (0, 0) L2
  measures "d9" distance of L2.end L0.start
  measures "d10" distance of L0.start L0.end
  measures "d11" distance of L6.start L6.end
hole "穴1" at (7, -5.5, 0) at (-7, -5.5, 0) direction (0, 0, 1) diameter 3.2 depth 14 tip angle 118 countersink diameter 6 countersink angle 90
